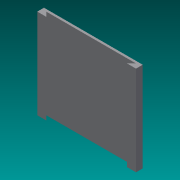
# Autodesk Inventor part: nano_enclosure_modular_sidelock
Saved by Autodesk Inventor 2015 (Build 190159000, 159)
## iProperties
Created: 2015-02-26
Part Number: nano_enclosure_modular_sidelock
Material: Generic
Document SubType Name: Modeling
Designer: Jeff
Density: 1 g/cm^3
Appearance: Default
Author: Jeff
Autodesk Inventor part; units mm, degrees
ref_plane "YZ Plane" through (0, 0, 0) normal (1, 0, 0) x (0, 1, 0)
ref_plane "XZ Plane" through (0, 0, 0) normal (0, 1, 0) x (-1, 0, 0)
ref_plane "XY Plane" through (0, 0, 0) normal (0, 0, 1) x (1, 0, 0)
sketch "Sketch1" plane through (0, 0, 0) normal (0, 0, 1) x (1, 0, 0)
  line L0 (0, 0) -> (55.88, 0)
  line L1 (55.88, 0) -> (55.88, 50.8)
  line L2 (55.88, 50.8) -> (0, 50.8)
  line L3 (0, 50.8) -> (0, 0)
  dimension "d0" = 55.88
  dimension "d1" = 50.8
  constraints: 8 end point, 2 parallel, 1 horizontal, 1 perpendicular
  measures "d0" distance of L2.end L1.end
  measures "d1" distance of L0.end L1.end
extrude "Extrusion1" add sketch "Sketch1" along normal blind 3.81
sketch "Sketch2" plane through (0, 0, 0) normal (0, -1, 0) x (1, 0, 0)
  line L0 (0, 3.81) -> (55.88, 3.81) projected
  line L1 (5.08, 3.81) -> (2.54, 1.27)
  line L2 (2.54, 1.27) -> (53.34, 1.27)
  line L3 (53.34, 1.27) -> (50.8, 3.81)
  line L4 (5.08, 3.81) -> (50.8, 3.81)
  line L5 (0, 0) -> (0, 3.81) projected
  line L6 (0, 0) -> (55.88, 0) projected
  line L7 (55.88, 0) -> (55.88, 3.81) projected
  dimension "d4" = 45
  dimension "d5" = 45
  dimension "d6" = 45.72
  dimension "d7" = 2.54
  dimension "d8" = 1.27
  dimension "d12" = 2.54
  dimension "d13" = 2.54
  constraints: 8 end point, 2 point on line, 1 collinear, 1 parallel
  measures "d4" angle of L2 L1
  measures "d5" angle of L2 L3
  measures "d6" distance of L3.end L1.start
  measures "d7" distance from line of L5 L1.end
  measures "d8" distance between parallel lines of L6 L2
  measures "d12" horizontal distance of L2.end L3.end
  measures "d13" distance from line of L7 L2.end
extrude "Extrusion2" cut sketch "Sketch2" against normal blind 50.8 contours L0 L3 L2 L1
body "Solid1"
